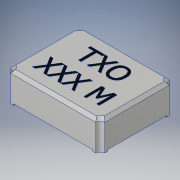
# Autodesk Inventor part: Crystal_TXO-3225
Saved by Autodesk Inventor 2018 (Build 220112000, 112)
## iProperties
Created: 2016-08-15
Part Number: Crystal_TXO-3225
Material: Aluminum 6061
Document SubType Name: Modeling
Designer: Bradley
Density: 2.7 g/cm^3
Appearance: Aluminum - Flat
Author: Bradley
Autodesk Inventor part; units mm, degrees
ref_plane "YZ Plane" through (0, 0, 0) normal (1, 0, 0) x (0, 1, 0)
ref_plane "XZ Plane" through (0, 0, 0) normal (0, 1, 0) x (-1, 0, 0)
ref_plane "XY Plane" through (0, 0, 0) normal (0, 0, 1) x (1, 0, 0)
sketch "Sketch1" plane through (0, 0, 0) normal (0, 1, 0) x (-1, 0, 0)
  line L0 (-1.6, 1.25) -> (1.6, 1.25)
  line L1 (1.6, 1.25) -> (1.6, -1.25)
  line L2 (1.6, -1.25) -> (-1.6, -1.25)
  line L3 (-1.6, -1.25) -> (-1.6, 1.25)
  line L4 (-1.6, 1.25) -> (1.6, -1.25) construction
  line L5 (1.6, 1.25) -> (-1.6, -1.25) construction
  arc A0 (1.6, -1.1) -> (1.45, -1.25) centre (1.6, -1.25) ccw
  arc A1 (-1.45, -1.25) -> (-1.6, -1.1) centre (-1.6, -1.25) ccw
  arc A2 (-1.6, 1.1) -> (-1.45, 1.25) centre (-1.6, 1.25) ccw
  arc A3 (1.45, 1.25) -> (1.6, 1.1) centre (1.6, 1.25) ccw
  point P0 (0, 0)
  dimension "d0" = 3.2
  dimension "d1" = 2.5
  dimension "d4" = 0.15
  constraints: 12 end point, 8 point on circle, 8 point on line, 4 centre point, 4 coincident, 3 equal radius, 2 midpoint, 2 parallel, 1 horizontal, 1 perpendicular
  measures "d0" distance of L1.end L2.end
  measures "d1" distance of L0.end L1.end
  measures "d4" radius of A0
extrude "Extrusion1" add sketch "Sketch1" along normal mid plane 0.95 contours L0 A3 L1 A0 L2 A1 L3 A2
chamfer "Chamfer1" distance 0.1 angle 45 8 edges at (0, 0.475, 1.25) (-1.4939, 0.475, 1.1439) (-1.6, 0.475, 0) (-1.4939, 0.475, -1.1439) (0, 0.475, -1.25) (1.4939, 0.475, -1.1439) (1.6, 0.475, 0) (1.4939, 0.475, 1.1439)
sketch "Sketch3" plane through (0, 0.475, 0) normal (0, 1, 0) x (1, 0, 0)
  line L0 (-1.3709, 1.15) -> (1.3709, 1.15) projected
  arc A0 (-1.5, 1.0209) -> (-1.3709, 1.15) centre (-1.6, 1.25) ccw projected
  line L1 (-1.5, -1.0209) -> (-1.5, 1.0209) projected
  arc A1 (-1.3709, -1.15) -> (-1.5, -1.0209) centre (-1.6, -1.25) ccw projected
  line L2 (1.3709, -1.15) -> (-1.3709, -1.15) projected
  arc A2 (1.5, -1.0209) -> (1.3709, -1.15) centre (1.6, -1.25) ccw projected
  line L3 (1.5, 1.0209) -> (1.5, -1.0209) projected
  arc A3 (1.3709, 1.15) -> (1.5, 1.0209) centre (1.6, 1.25) ccw projected
  line L4 (1.5, 1.0209) -> (1.5, -1.0209) construction
  line L5 (1.5, 0.1868) -> (-1.5, 0.1868) construction
  line L6 (-0.5716, 0.1868) -> (-0.5716, 0.7158)
  line L7 (-0.5716, 0.7158) -> (-0.7729, 0.7158)
  line L8 (-0.7729, 0.7158) -> (-0.7729, 0.7868)
  line L9 (-0.7729, 0.7868) -> (-0.2905, 0.7868)
  line L10 (-0.2905, 0.7868) -> (-0.2905, 0.7158)
  line L11 (-0.2905, 0.7158) -> (-0.4918, 0.7158)
  line L12 (-0.4918, 0.7158) -> (-0.4918, 0.1868)
  line L13 (-0.4918, 0.1868) -> (-0.5716, 0.1868)
  line L14 (0.1855, 0.1868) -> (0.0941, 0.1868)
  line L15 (0.0941, 0.1868) -> (-0.0518, 0.426)
  line L16 (-0.0518, 0.426) -> (-0.2006, 0.1868)
  line L17 (-0.2006, 0.1868) -> (-0.2866, 0.1868)
  line L18 (-0.2866, 0.1868) -> (-0.0955, 0.4872)
  line L19 (-0.0955, 0.4872) -> (-0.2808, 0.7868)
  line L20 (-0.2808, 0.7868) -> (-0.1894, 0.7868)
  line L21 (-0.1894, 0.7868) -> (-0.0464, 0.5519)
  line L22 (-0.0464, 0.5519) -> (0.0994, 0.7868)
  line L23 (0.0994, 0.7868) -> (0.1855, 0.7868)
  line L24 (0.1855, 0.7868) -> (-0.0022, 0.4911)
  line L25 (-0.0022, 0.4911) -> (0.1855, 0.1868)
  spline S0 degree 2 poles (0.6741, 0.7182) (0.7082, 0.6783) (0.7461, 0.5616) (0.7461, 0.4868) knots 0 0 0 1 2 2 2
  spline S1 degree 2 poles (0.7461, 0.4868) (0.7461, 0.4138) (0.7092, 0.2957) (0.6741, 0.2558) knots 0 0 0 1 2 2 2
  spline S2 degree 2 poles (0.6741, 0.2558) (0.6372, 0.214) (0.5395, 0.1741) (0.4806, 0.1741) knots 0 0 0 1 2 2 2
  spline S3 degree 2 poles (0.4806, 0.1741) (0.4199, 0.1741) (0.3226, 0.2154) (0.2871, 0.2558) knots 0 0 0 1 2 2 2
  spline S4 degree 2 poles (0.2871, 0.2558) (0.2526, 0.2957) (0.2156, 0.4129) (0.2156, 0.4868) knots 0 0 0 1 2 2 2
  spline S5 degree 2 poles (0.2156, 0.4868) (0.2156, 0.5621) (0.2531, 0.6769) (0.2876, 0.7182) knots 0 0 0 1 2 2 2
  spline S6 degree 2 poles (0.2876, 0.7182) (0.3226, 0.7581) (0.4203, 0.7994) (0.4806, 0.7994) knots 0 0 0 1 2 2 2
  spline S7 degree 2 poles (0.4806, 0.7994) (0.5419, 0.7994) (0.6401, 0.7566) (0.6741, 0.7182) knots 0 0 0 1 2 2 2
  spline S8 degree 2 poles (0.663, 0.4868) (0.663, 0.5461) (0.6372, 0.638) (0.6139, 0.6681) knots 0 0 0 1 2 2 2
  spline S9 degree 2 poles (0.6139, 0.6681) (0.59, 0.6992) (0.5229, 0.7304) (0.4811, 0.7304) knots 0 0 0 1 2 2 2
  spline S10 degree 2 poles (0.4811, 0.7304) (0.4378, 0.7304) (0.3727, 0.7002) (0.3479, 0.6681) knots 0 0 0 1 2 2 2
  spline S11 degree 2 poles (0.3479, 0.6681) (0.3241, 0.6375) (0.2988, 0.5451) (0.2988, 0.4868) knots 0 0 0 1 2 2 2
  spline S12 degree 2 poles (0.2988, 0.4868) (0.2988, 0.3686) (0.398, 0.2432) (0.4811, 0.2432) knots 0 0 0 1 2 2 2
  spline S13 degree 2 poles (0.4811, 0.2432) (0.5643, 0.2432) (0.663, 0.3686) (0.663, 0.4868) knots 0 0 0 1 2 2 2
  line L26 (-0.6897, -0.7914) -> (-0.7811, -0.7914)
  line L27 (-0.7811, -0.7914) -> (-0.927, -0.5522)
  line L28 (-0.927, -0.5522) -> (-1.0758, -0.7914)
  line L29 (-1.0758, -0.7914) -> (-1.1618, -0.7914)
  line L30 (-1.1618, -0.7914) -> (-0.9707, -0.4909)
  line L31 (-0.9707, -0.4909) -> (-1.156, -0.1914)
  line L32 (-1.156, -0.1914) -> (-1.0646, -0.1914)
  line L33 (-1.0646, -0.1914) -> (-0.9216, -0.4263)
  line L34 (-0.9216, -0.4263) -> (-0.7758, -0.1914)
  line L35 (-0.7758, -0.1914) -> (-0.6897, -0.1914)
  line L36 (-0.6897, -0.1914) -> (-0.8774, -0.487)
  line L37 (-0.8774, -0.487) -> (-0.6897, -0.7914)
  line L38 (-0.2108, -0.7914) -> (-0.3022, -0.7914)
  line L39 (-0.3022, -0.7914) -> (-0.4481, -0.5522)
  line L40 (-0.4481, -0.5522) -> (-0.5968, -0.7914)
  line L41 (-0.5968, -0.7914) -> (-0.6829, -0.7914)
  line L42 (-0.6829, -0.7914) -> (-0.4918, -0.4909)
  line L43 (-0.4918, -0.4909) -> (-0.6771, -0.1914)
  line L44 (-0.6771, -0.1914) -> (-0.5857, -0.1914)
  line L45 (-0.5857, -0.1914) -> (-0.4427, -0.4263)
  line L46 (-0.4427, -0.4263) -> (-0.2968, -0.1914)
  line L47 (-0.2968, -0.1914) -> (-0.2108, -0.1914)
  line L48 (-0.2108, -0.1914) -> (-0.3985, -0.487)
  line L49 (-0.3985, -0.487) -> (-0.2108, -0.7914)
  line L50 (0.2682, -0.7914) -> (0.1767, -0.7914)
  line L51 (0.1767, -0.7914) -> (0.0309, -0.5522)
  line L52 (0.0309, -0.5522) -> (-0.1179, -0.7914)
  line L53 (-0.1179, -0.7914) -> (-0.204, -0.7914)
  line L54 (-0.204, -0.7914) -> (-0.0129, -0.4909)
  line L55 (-0.0129, -0.4909) -> (-0.1981, -0.1914)
  line L56 (-0.1981, -0.1914) -> (-0.1067, -0.1914)
  line L57 (-0.1067, -0.1914) -> (0.0362, -0.4263)
  line L58 (0.0362, -0.4263) -> (0.1821, -0.1914)
  line L59 (0.1821, -0.1914) -> (0.2682, -0.1914)
  line L60 (0.2682, -0.1914) -> (0.0805, -0.487)
  line L61 (0.0805, -0.487) -> (0.2682, -0.7914)
  line L62 (1.1045, -0.7914) -> (1.0247, -0.7914)
  line L63 (1.0247, -0.7914) -> (1.0247, -0.2746)
  line L64 (1.0247, -0.2746) -> (0.8682, -0.6261)
  line L65 (0.8682, -0.6261) -> (0.8195, -0.6261)
  line L66 (0.8195, -0.6261) -> (0.6644, -0.2746)
  line L67 (0.6644, -0.2746) -> (0.6644, -0.7914)
  line L68 (0.6644, -0.7914) -> (0.59, -0.7914)
  line L69 (0.59, -0.7914) -> (0.59, -0.1914)
  line L70 (0.59, -0.1914) -> (0.6989, -0.1914)
  line L71 (0.6989, -0.1914) -> (0.8487, -0.5255)
  line L72 (0.8487, -0.5255) -> (0.9936, -0.1914)
  line L73 (0.9936, -0.1914) -> (1.1045, -0.1914)
  line L74 (1.1045, -0.1914) -> (1.1045, -0.7914)
  point P0 (0, 0)
  constraints: 2 end point, 2 point on line, 1 horizontal, 1 perpendicular
extrude "Extrusion3" add sketch "Sketch3" along normal blind 0.01 contours L6 L7 L8 L9 L10 L11 L12 L13 | L14 L15 L16 L17 L18 L19 L20 L21 L22 L23 L24 L25 | S0 S1 S2 S3 S4 S5 S6 S7 | L26 L27 L28 L29 L30 L31 L32 L33 L34 L35 L36 L37 | L38 L39 L40 L41 L42 L43 L44 L45 L46 L47 L48 L49 | L50 L51 L52 L53 L54 L55 L56 L57 L58 L59 L60 L61 | L62 L63 L64 L65 L66 L67 L68 L69 L70 L71 L72 L73 L74
sketch "Sketch4" plane through (0, -0.475, 0) normal (0, -1, 0) x (1, 0, 0)
  line L0 (-1.6, 1.1) -> (-1.6, -1.1) projected
  arc A0 (-1.45, -1.25) -> (-1.6, -1.1) centre (-1.6, -1.25) ccw projected
  line L1 (-1.45, -1.25) -> (1.45, -1.25) projected
  arc A1 (1.6, -1.1) -> (1.45, -1.25) centre (1.6, -1.25) ccw projected
  line L2 (1.6, -1.1) -> (1.6, 1.1) projected
  arc A2 (1.45, 1.25) -> (1.6, 1.1) centre (1.6, 1.25) ccw projected
  line L3 (1.45, 1.25) -> (-1.45, 1.25) projected
  arc A3 (-1.6, 1.1) -> (-1.45, 1.25) centre (-1.6, 1.25) ccw projected
  line L4 (1.35, 1.25) -> (1.35, 1.19)
  line L5 (1.35, 1.19) -> (0.94, 1.19)
  line L6 (0.94, 1.19) -> (0.94, 0.35)
  line L7 (0.94, 0.35) -> (1.54, 0.35)
  line L8 (1.54, 0.35) -> (1.54, 1)
  line L9 (1.54, 1) -> (1.6, 1)
  line L10 (-1.6, -1.1) -> (-1.6, 1.1) projected
  line L11 (-1.6, 1) -> (-1.54, 1)
  line L12 (-1.54, 1) -> (-1.54, 0.35)
  line L13 (-1.54, 0.35) -> (-0.94, 0.35)
  line L14 (-0.94, 0.35) -> (-0.94, 1.19)
  line L15 (-0.94, 1.19) -> (-1.35, 1.19)
  line L16 (-1.35, 1.19) -> (-1.35, 1.25)
  line L17 (1.45, -1.25) -> (-1.45, -1.25) projected
  line L18 (-1.35, -1.25) -> (-1.35, -1.19)
  line L19 (-1.35, -1.19) -> (-0.94, -1.19)
  line L20 (-0.94, -1.19) -> (-0.94, -0.35)
  line L21 (-0.94, -0.35) -> (-1.54, -0.35)
  line L22 (-1.54, -0.35) -> (-1.54, -1)
  line L23 (-1.54, -1) -> (-1.6, -1)
  line L24 (1.6, -1) -> (1.54, -1)
  line L25 (1.54, -1) -> (1.54, -0.35)
  line L26 (1.54, -0.35) -> (0.94, -0.35)
  line L27 (0.94, -0.35) -> (0.94, -1.19)
  line L28 (0.94, -1.19) -> (1.35, -1.19)
  line L29 (1.35, -1.19) -> (1.35, -1.25)
  point P0 (0, 0)
  dimension "d20" = 0.84
  dimension "d21" = 0.6
  dimension "d22" = 1.88
  dimension "d23" = 0.25
  dimension "d24" = 0.25
  constraints: 48 end point, 20 point on line, 15 perpendicular, 7 equal length, 6 collinear, 1 horizontal, 1 parallel, 1 vertical
  measures "d20" distance of L5.end L6.end
  measures "d21" distance of L6.end L7.end
  measures "d22" distance between parallel lines of L14 L6
  measures "d23" distance between parallel lines of L4 L2
  measures "d24" distance between parallel lines of L9 L3
extrude "Extrusion5" add sketch "Sketch4" along normal blind 0.05 contours A3 L3 L16 L15 L14 L13 L12 L11 L0 | L23 L22 L21 L20 L19 L18 L1 A0 L0 | L3 A2 L2 L9 L8 L7 L6 L5 L4 | L29 L28 L27 L26 L25 L24 L2 A1 L1
equation "\"d24\" = d23"
body "Solid1"
